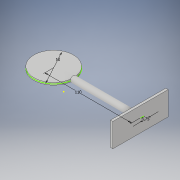
# Autodesk Inventor part: Kreisverkehrsschild_Teil_Unten
Saved by Autodesk Inventor 2019.5 (Build 235369000, 369)
## iProperties
Created: 2021-09-30
Part Number: Kreisverkehrsschild_Teil_Unten
Material: Generisch
Document SubType Name: Modeling
Designer: mritt
Density: 1 g/cm^3
Appearance: Vorgabe
Author: mritt
Autodesk Inventor part; units mm, degrees
ref_plane "YZ Plane" through (0, 0, 0) normal (1, 0, 0) x (0, 1, 0)
ref_plane "XZ Plane" through (0, 0, 0) normal (0, 1, 0) x (-1, 0, 0)
ref_plane "XY Plane" through (0, 0, 0) normal (0, 0, 1) x (1, 0, 0)
sketch "Skizze1" plane through (0, 0, 0) normal (0, 1, 0) x (-1, 0, 0)
  circle A0 centre (32.7504, -19.9257) radius 25
  line L0 (32.7504, -19.9257) -> (-77.2496, -19.9257)
  line L1 (-77.2496, -19.9257) -> (-77.2496, -23.6757)
  line L2 (-77.2496, -23.6757) -> (8.0333, -23.6757)
  line L3 (8.0333, -23.6757) -> (8.0333, -19.9257)
  point P0 (0, 0)
  dimension "d4" = 50
  dimension "d9" = 110
  dimension "d10" = 3.75
  constraints: 8 end point, 2 horizontal, 1 perpendicular, 1 point on line, 1 vertical, 3 other
  measures "d9" distance of L0.start L0.end
  measures "d10" distance of L0.end L1.end
extrude "Extrusion1" add sketch "Skizze1" along normal blind 1.5 and the other way blind 1.5 contours L3 L0 A0 | A0 L0 L3
revolve "Umdrehung1" add sketch "Skizze1" angle 360 about axis through (-32.7504, 0, -19.9257) along (1, 0, 0) picked at (7.9809, -22.0108) contours L2 L1 L0 A0 | A0 L0 L3
sketch "Skizze2" plane through (77.2496, 0, -19.9257) normal (1, 0, 0) x (0, 0, -1)
  line L0 (35, -16.5) -> (-35, -16.5)
  line L1 (-35, -16.5) -> (-35, 13.5)
  line L2 (-35, 13.5) -> (35, 13.5)
  line L3 (35, 13.5) -> (35, -16.5)
  line L4 (-25, -1.5) -> (25, -1.5) projected
  line L5 (35, -16.5) -> (-35, 13.5) construction
  line L6 (-35, -16.5) -> (35, 13.5) construction
  point P0 (-19.9257, 0)
  point P1 (0, -1.5)
  point P2 (-3.75, 0)
  point P3 (3.75, 0)
  dimension "d14" = 70
  dimension "d15" = 30
  constraints: 12 end point, 2 midpoint, 2 parallel, 1 horizontal, 1 perpendicular, 2 other
  measures "d14" distance of L1.end L2.end
  measures "d15" distance of L0.end L1.end
extrude "Extrusion2" add sketch "Skizze2" against normal blind 3
